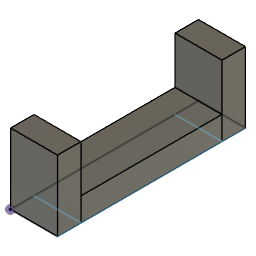
bridge (Autodesk Fusion 360 design; units mm, degrees)
part number: 2026-06-19-19-02-43-658
Autodesk Fusion 360 part; units mm, degrees
sketch "Szkic1" plane through (0, 0, 0) normal (0, 0, 1) x (1, 0, 0)
  line L0 (0, 0) -> (10, 0)
  line L1 (10, 0) -> (10, 40)
  line L2 (0, 0) -> (0, 40)
  line L3 (0, 40) -> (10, 40)
  line L4 (0, 5) -> (10, 5)
  line L5 (0, 35) -> (10, 35)
  dimension "d3" = 40
  constraint coincident L0.start L2.start
  constraint horizontal L0
  constraint perpendicular L0 L1
  constraint perpendicular L0 L2
  constraint perpendicular L1 L3
  constraint coincident L2 L4.start
  constraint coincident L1 L4.end
  constraint perpendicular L1 L4
  constraint coincident L2 L5.start
  constraint coincident L1 L5.end
  constraint perpendicular L1 L5
  measures "d3" distance of L0.start L2.end
extrude "Wyciągnięcie proste1" add sketch "Szkic1" along normal blind 15 contours L0 L1 L2 L4 | L1 L2 L3 L5 makes body 1 at (3.3333, 40, 5) makes body 2 at (3.3333, 5, 5)
extrude "Wyciągnięcie proste2" add sketch "Szkic1" along normal blind 5 separate body contours L1 L2 L4 L5 makes body 3
